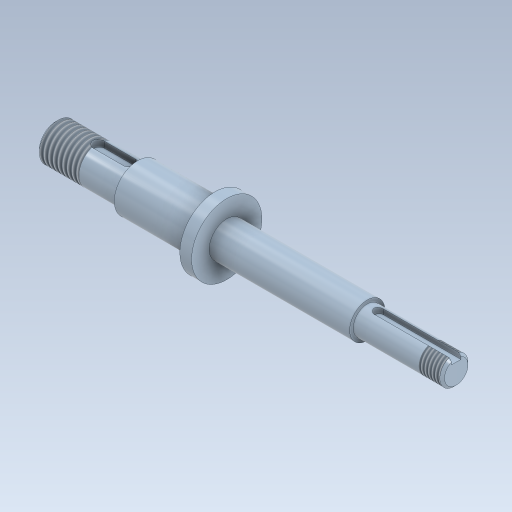
# Autodesk Inventor part: Pump-Motor-CW-Rotation:Shaft
Saved by Autodesk Inventor 2024.2 (Build 282272000, 272)
## iProperties
Created: 2025-06-16
Material: Steel, Alloy
Document SubType Name: Modeling
Density: 7.73 g/cm^3
Appearance: Steel Blue
Designer: cw
Author: cw
Autodesk Inventor part; units mm, degrees
ref_plane "YZ Plane" through (0, 0, 0) normal (1, 0, 0) x (0, 1, 0)
ref_plane "XZ Plane" through (0, 0, 0) normal (0, 1, 0) x (-1, 0, 0)
sketch "Sketch1" plane through (0, 0, 0) normal (0, 0, 1) x (1, 0, 0)
  line L0 (-85.5, 0) -> (85.5, 0)
  line L1 (85.5, 0) -> (85.5, 6)
  line L2 (85.5, 6) -> (47.5, 6)
  line L3 (47.5, 6) -> (47.5, 7.5)
  line L4 (47.5, 7.5) -> (-12.5, 7.5)
  line L5 (-12.5, 7.5) -> (-12.5, 15)
  line L6 (-12.5, 15) -> (-17.5, 15)
  line L7 (-17.5, 15) -> (-17.5, 10)
  line L8 (-17.5, 10) -> (-50.5, 10)
  line L9 (-85.5, 0) -> (-85.5, 8)
  line L10 (-85.5, 8) -> (-50.5, 8)
  line L11 (-50.5, 10) -> (-50.5, 8)
  point P0 (0, 0)
  point P1 (0, 0)
  dimension "d8" = 12
  dimension "d9" = 15
  dimension "d10" = 30
  dimension "d11" = 20
  dimension "d12" = 98
  dimension "d13" = 5
  dimension "d14" = 60
  dimension "d15" = 33
  dimension "d16" = 16
  dimension "d43" = 68
  constraints: 24 end point, 8 perpendicular, 3 vertical, 1 coincident, 1 horizontal, 1 midpoint
  measures "d8" diameter of L2 L0
  measures "d9" diameter of L4 L0
  measures "d10" diameter of L6 L0
  measures "d11" diameter of L8 L0
  measures "d12" distance between parallel lines of L1 L5
  measures "d13" distance of L5.end L6.end
  measures "d14" distance between parallel lines of L3 L5
  measures "d15" distance from line of L7 L8.end
  measures "d16" diameter of L10 L0
  measures "d43" distance between parallel lines of L7 L9
revolve "Revolution1" add sketch "Sketch1" angle 360 about axis through (-85.5, 0, 0) along (1, 0, 0)
thread "Thread1" size "M12x1.5" class "6g" standard "ISO Metric profile" length 10
chamfer "Chamfer1" distance 1 angle 45 2 edges at (85.5, -6, 0) (-85.5, -8, 0)
sketch "Sketch4" plane through (85.5, 0, 0) normal (1, 0, 0) x (0, 0, -1)
  circle A0 centre (0, 0) radius 6 projected
  line L0 (-5.6569, -2) -> (-3.5, -2)
  line L1 (-3.5, -2) -> (-3.5, 2)
  line L2 (-3.5, 2) -> (-5.6569, 2)
  point P0 (0, 0)
  dimension "d35" = 9.5
  dimension "d36" = 4
  constraints: 6 end point, 2 perpendicular, 2 point on circle, 1 horizontal, 1 parallel
  measures "d36" distance between parallel lines of L2 L0
extrude "Extrusion3" cut sketch "Sketch4" against normal blind 35 contours L2 L1 L0 A0 picked at (-4.3205, -0.2261)
full round fillet "Full Round Fillet1" first side at (73.5, -2, 4.219) centre faces at (50.5, 0.2261, 4.3205) second side at (73.5, 2, 4.219)
thread "Thread2" size "M16x2" class "6g" standard "ANSI Metric M Profile" length 17
ref_plane "Work Plane2" through (-68, 0, 8) normal (0, 0, 1) x (1, 0, 0)
sketch "Sketch3" plane through (-68, 0, 8) normal (0, 0, 1) x (1, 0, 0)
  line L0 (14, -2.5) -> (1, -2.5)
  arc A0 (1, 2.5) -> (1, -2.5) centre (1, 0) ccw
  line L1 (1, 2.5) -> (14, 2.5)
  arc A1 (14, -2.5) -> (14, 2.5) centre (14, 0) ccw
  line L2 (-51.7, 0) -> (187.7, 0) projected
  line L3 (-17.5, -7) -> (-17.5, 7) projected
  point P0 (68, 0)
  point P1 (16.5, 0)
  point P2 (-1.5, 0)
  dimension "d40" = 18
  dimension "d41" = 5
  dimension "d42" = 16
  constraints: 6 point on circle, 4 end point, 4 tangent, 2 centre point, 2 point on line, 1 parallel
  measures "d40" distance of point (-1.5, 0) point (16.5, 0)
  measures "d41" distance between parallel lines of L0 L1
  measures "d42" distance from line of point (-1.5, 0) L3
extrude "Extrusion2" cut sketch "Sketch3" against normal blind 3
body "Solid1"
